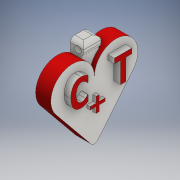
# Autodesk Inventor part: Part1
Saved by Autodesk Inventor 2016 (Build 200138000, 138)
## iProperties
Created: 2016-02-03
Part Number: Part1
Material: Generic
Document SubType Name: Modeling
Designer: TimB
Density: 1 g/cm^3
Appearance: White
Author: TimB
Autodesk Inventor part; units mm, degrees
ref_plane "YZ Plane" through (0, 0, 0) normal (1, 0, 0) x (0, 1, 0)
ref_plane "XZ Plane" through (0, 0, 0) normal (0, 1, 0) x (-1, 0, 0)
ref_plane "XY Plane" through (0, 0, 0) normal (0, 0, 1) x (1, 0, 0)
sketch "Sketch1" plane through (0, 0, 0) normal (0, 1, 0) x (-1, 0, 0)
  line L0 (-18, 0) -> (3.6652, 17.7376)
  line L1 (-18, 0) -> (3.6652, -17.7376)
  arc A0 (10, 0) -> (3.6652, 17.7376) centre (10, 10) ccw
  arc A1 (3.6652, -17.7376) -> (10, 0) centre (10, -10) ccw
  point P0 (0, 0)
  dimension "d4" = 18
  constraints: 4 end point, 4 point on circle, 3 tangent, 2 centre point
  measures "d4" distance of point (0, 0) L0.start
extrude "Extrusion1" add sketch "Sketch1" along normal blind 7
sketch "Sketch2" plane through (0, 7, 0) normal (0, 1, 0) x (1, 0, 0)
  line L0 (-3.6652, -17.7376) -> (18, 0) projected
  line L1 (18, 0) -> (-3.6652, 17.7376) projected
  line L2 (-3.6652, -17.7376) -> (-3.6652, 17.7376)
  spline S0 degree 2 poles (-3.4318, -9.1343) (-3.4318, -11.2931) (-6.6992, -13.8312) (-9.6554, -13.8312) knots 0 0 0 1 2 2 2
  spline S1 degree 2 poles (-9.6554, -13.8312) (-12.5047, -13.8312) (-15.8985, -11.2834) (-15.8985, -9.1343) knots 0 0 0 1 2 2 2
  spline S2 degree 2 poles (-15.8985, -9.1343) (-15.8985, -8.5605) (-15.7332, -7.6464) (-15.5971, -7.2283) knots 0 0 0 1 2 2 2
  spline S3 degree 2 poles (-15.5971, -7.2283) (-15.4707, -6.8977) (-15.0525, -6.1197) (-14.8969, -5.8863) knots 0 0 0 1 2 2 2
  line L3 (-14.8969, -5.8863) -> (-12.0379, -5.8863)
  line L4 (-12.0379, -5.8863) -> (-12.0379, -6.1294)
  spline S4 degree 2 poles (-12.0379, -6.1294) (-12.2324, -6.3045) (-12.777, -6.8296) (-13.0298, -7.1699) knots 0 0 0 1 2 2 2
  spline S5 degree 2 poles (-13.0298, -7.1699) (-13.2924, -7.5006) (-13.6522, -8.3077) (-13.6522, -8.7453) knots 0 0 0 1 2 2 2
  spline S6 degree 2 poles (-13.6522, -8.7453) (-13.6522, -9.2607) (-13.2438, -10.1359) (-12.7284, -10.5249) knots 0 0 0 1 2 2 2
  spline S7 degree 2 poles (-12.7284, -10.5249) (-12.2713, -10.8847) (-10.7057, -11.3417) (-9.6457, -11.3417) knots 0 0 0 1 2 2 2
  spline S8 degree 2 poles (-9.6457, -11.3417) (-8.5274, -11.3417) (-7.0007, -10.8652) (-6.5339, -10.4763) knots 0 0 0 1 2 2 2
  spline S9 degree 2 poles (-6.5339, -10.4763) (-6.0768, -10.1067) (-5.6781, -9.1829) (-5.6781, -8.7259) knots 0 0 0 1 2 2 2
  spline S10 degree 2 poles (-5.6781, -8.7259) (-5.6781, -8.2494) (-6.0768, -7.3936) (-6.3199, -7.0921) knots 0 0 0 1 2 2 2
  spline S11 degree 2 poles (-6.3199, -7.0921) (-6.5631, -6.7712) (-7.0784, -6.285) (-7.2827, -6.1002) knots 0 0 0 1 2 2 2
  line L5 (-7.2827, -6.1002) -> (-7.2827, -5.8863)
  line L6 (-7.2827, -5.8863) -> (-4.4626, -5.8863)
  spline S12 degree 2 poles (-4.4626, -5.8863) (-4.307, -6.1489) (-3.918, -6.849) (-3.7819, -7.2088) knots 0 0 0 1 2 2 2
  spline S13 degree 2 poles (-3.7819, -7.2088) (-3.6068, -7.6659) (-3.4318, -8.4438) (-3.4318, -9.1343) knots 0 0 0 1 2 2 2
  line L7 (-3.6652, 9.0176) -> (-13.3799, 9.0176)
  line L8 (-13.3799, 9.0176) -> (-13.3799, 6.1878)
  line L9 (-13.3799, 6.1878) -> (-15.6652, 6.1878)
  line L10 (-15.6652, 6.1878) -> (-15.6652, 14.2591)
  line L11 (-15.6652, 14.2591) -> (-13.3799, 14.2591)
  line L12 (-13.3799, 14.2591) -> (-13.3799, 11.4293)
  line L13 (-13.3799, 11.4293) -> (-3.6652, 11.4293)
  line L14 (-3.6652, 11.4293) -> (-3.6652, 9.0176)
  point P0 (0, 0)
  constraints: 2 end point, 2 vertical
sketch "Sketch3" plane through (0, 0, 0) normal (0, -1, 0) x (1, 0, 0)
  arc A0 (-10, 0) -> (-3.6652, -17.7376) centre (-10, -10) ccw projected
  arc A1 (-3.6652, 17.7376) -> (-10, 0) centre (-10, 10) ccw projected
  arc A2 (-10, 0) -> (-3.6652, -17.7376) centre (-10, -10) ccw projected
  line L0 (-18, -4) -> (-18, 4)
  point P0 (0, 0)
  point P1 (-20, 10)
  constraints: 3 point on circle, 2 end point
extrude "Extrusion5" add sketch "Sketch3" against normal blind 5
sketch "Sketch5" plane through (-18, 0, -4) normal (-1, 0, 0) x (0, 0, 1)
  line L0 (0, 5) -> (8, 5) projected
  line L1 (8, 0) -> (0, 0) projected
  line L2 (8, 5) -> (8, 0) projected
  line L3 (0, 5) -> (8, 5) projected
  line L4 (0, 0) -> (0, 5) projected
  point P0 (4, 0)
extrude "Extrusion6" add sketch "Sketch5" along normal blind 6
sketch "Sketch7" plane through (0, 5, 0) normal (0, 1, 0) x (1, 0, 0)
  line L0 (-18, -4) -> (-24, -4) projected
  line L1 (-24, 4) -> (-24, -4) projected
  line L2 (-24, -4) -> (-24, 4)
  line L3 (-24, 4) -> (-19, 4)
  line L4 (-19, 4) -> (-19, -4)
  line L5 (-19, -4) -> (-24, -4)
  point P0 (0, 0)
  dimension "d20" = 5
  constraints: 8 end point, 3 equal length, 1 perpendicular
  measures "d20" distance of L1.start L3.end
extrude "Extrusion7" add sketch "Sketch7" along normal blind 1
sketch "Sketch8" plane through (-18, 0, -4) normal (0, 0, -1) x (-1, 0, 0)
  line L0 (6, 0) -> (3, 0)
  line L1 (3, 0) -> (3, 3.5)
  line L2 (3, 3.5) -> (6, 3.5)
  line L3 (6, 3.5) -> (6, 0)
  point P0 (-18, 0)
  dimension "d23" = 3
  dimension "d24" = 3.5
  constraints: 8 end point, 2 parallel, 1 horizontal, 1 perpendicular
  measures "d23" distance of L1.end L2.end
  measures "d24" distance of L0.end L1.end
hole "Hole1" at (-21, 3.5, -4) direction (0, 0, 1) diameter 3 depth 8 tip angle 118
fillet "Fillet1" radius 2 4 edges at (-19, 6, 0) (-24, 6, 0) (-24, 3, -4) (-24, 3, 4)
fillet "Fillet3" radius 2 1 edges at (18, 3.5, 0)
extrude "Extrusion8" add sketch "Sketch2" along normal blind 3 contours S0 S1 S2 S3 L3 L4 S4 S5 S6 S7 S8 S9 S10 S11 L5 L6 S12 S13 L2 | L2 S13 S0 | L2 L7 L8 L9 L10 L11 L12 L13
sketch "Sketch9" plane through (0, 7, 0) normal (0, 1, 0) x (1, 0, 0)
  point P0 (0, 0)
sketch "Sketch10" plane through (0, 7, 0) normal (0, 1, 0) x (1, 0, 0)
  line L0 (-3.6652, -17.7376) -> (16.1098, -1.5475) projected
  line L1 (3.7822, -11.6403) -> (3.7822, 11.6403)
  line L2 (16.1098, 1.5475) -> (-3.6652, 17.7376) projected
  line L3 (0.9491, 3.4587) -> (0.9491, 0.7099)
  line L4 (0.9491, 0.7099) -> (3.6785, 0.7099)
  line L5 (3.6785, 0.7099) -> (3.6785, -0.7099)
  line L6 (3.6785, -0.7099) -> (0.9491, -0.7099)
  line L7 (0.9491, -0.7099) -> (0.9491, -3.4587)
  line L8 (0.9491, -3.4587) -> (-0.4382, -3.4587)
  line L9 (-0.4382, -3.4587) -> (-0.4382, -0.7099)
  line L10 (-0.4382, -0.7099) -> (-3.1675, -0.7099)
  line L11 (-3.1675, -0.7099) -> (-3.1675, 0.7099)
  line L12 (-3.1675, 0.7099) -> (-0.4382, 0.7099)
  line L13 (-0.4382, 0.7099) -> (-0.4382, 3.4587)
  line L14 (-0.4382, 3.4587) -> (0.9491, 3.4587)
  point P0 (0, 0)
  constraints: 2 end point, 2 point on line, 2 vertical
extrude "Extrusion9" add sketch "Sketch10" along normal blind 1.5
body "Solid1"
